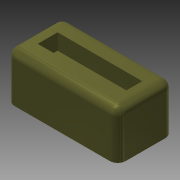
# Autodesk Inventor part: cover
Saved by Autodesk Inventor 2014 SP1 (Build 180222100, 222)
## iProperties
Created: 2016-10-06
Part Number: cover
Material: Titanium
Document SubType Name: Modeling
Designer: tguillod
Density: 4.51 g/cm^3
Appearance: Titanium
Author: tguillod
Autodesk Inventor part; units mm, degrees
ref_plane "YZ Plane" through (0, 0, 0) normal (1, 0, 0) x (0, 1, 0)
ref_plane "XZ Plane" through (0, 0, 0) normal (0, 1, 0) x (-1, 0, 0)
ref_plane "XY Plane" through (0, 0, 0) normal (0, 0, 1) x (1, 0, 0)
sketch "Sketch1" plane through (0, 0, 0) normal (0, 0, 1) x (1, 0, 0)
  line L0 (0, 0) -> (14, 0)
  line L1 (14, 0) -> (14, 7)
  line L2 (14, 7) -> (0, 7)
  line L3 (0, 7) -> (0, 0)
  dimension "d2" = 14
  dimension "d3" = 7
  constraints: 8 end point, 2 parallel, 1 horizontal, 1 perpendicular
  measures "d2" distance of L1.end L2.end
  measures "d3" distance of L0.end L1.end
extrude "Extrusion1" add sketch "Sketch1" along normal blind 6
sketch "Sketch2" plane through (0, 0, 6) normal (0, 0, 1) x (1, 0, 0)
  line L0 (0, 7) -> (14, 0) construction
  line L1 (0, 0) -> (14, 7) construction
  line L2 (1.67, 4.75) -> (12.33, 4.75)
  line L3 (12.33, 4.75) -> (12.33, 2.25)
  line L4 (12.33, 2.25) -> (1.67, 2.25)
  line L5 (1.67, 2.25) -> (1.67, 4.75)
  line L6 (1.67, 4.75) -> (12.33, 2.25) construction
  line L7 (12.33, 4.75) -> (1.67, 2.25) construction
  point P0 (7, 3.5)
  dimension "d4" = 2.5
  dimension "d5" = 10.66
  constraints: 16 end point, 3 midpoint, 2 parallel, 1 horizontal, 1 perpendicular
  measures "d4" distance of L2.end L3.end
  measures "d5" distance of L2.start L2.end
extrude "Extrusion3" cut sketch "Sketch2" against normal blind 2
sketch "Sketch3" plane through (0, 0, 4) normal (0, 0, 1) x (1, 0, 0)
  line L0 (1.67, 4.75) -> (12.33, 4.75) projected
  line L1 (1.67, 2.25) -> (1.67, 4.75) projected
  line L2 (12.33, 2.25) -> (1.67, 2.25) projected
  line L3 (12.33, 4.75) -> (12.33, 2.25) projected
  line L4 (2.67, 3.75) -> (11.33, 3.75)
  line L5 (11.33, 3.75) -> (11.33, 3.25)
  line L6 (11.33, 3.25) -> (2.67, 3.25)
  line L7 (2.67, 3.25) -> (2.67, 3.75)
  point P0 (0, 0)
  dimension "d10" = 1
  dimension "d11" = 1
  dimension "d12" = 1
  dimension "d13" = 1
  constraints: 8 end point, 2 parallel, 1 horizontal, 1 perpendicular
  measures "d10" distance between parallel lines of L1 L7
  measures "d11" distance between parallel lines of L3 L5
  measures "d12" distance between parallel lines of L0 L4
  measures "d13" distance between parallel lines of L6 L2
extrude "Extrusion4" cut sketch "Sketch3" against normal blind 4 contours L4 L5 L6 L7
sketch "Sketch4" plane through (0, 0, 0) normal (0, 0, -1) x (-1, 0, 0)
  line L0 (-2.67, 3.75) -> (-2.67, 3.25) projected
  line L1 (-2.67, 3.25) -> (-11.33, 3.25) projected
  line L2 (-11.33, 3.25) -> (-11.33, 3.75) projected
  line L3 (-11.33, 3.75) -> (-2.67, 3.75) projected
  line L4 (0, 0) -> (-14, 0) projected
  line L5 (0, 7) -> (0, 0) projected
  line L6 (-14, 7) -> (0, 7) projected
  line L7 (-14, 0) -> (-14, 7) projected
  line L8 (-13, 6) -> (-1, 6)
  line L9 (-1, 6) -> (-1, 1)
  line L10 (-1, 1) -> (-13, 1)
  line L11 (-13, 1) -> (-13, 6)
  dimension "d16" = 1
  dimension "d17" = 1
  dimension "d18" = 1
  dimension "d19" = 1
  constraints: 8 end point, 2 parallel, 1 horizontal, 1 perpendicular
  measures "d16" distance between parallel lines of L6 L8
  measures "d17" distance between parallel lines of L10 L4
  measures "d18" distance between parallel lines of L11 L7
  measures "d19" distance between parallel lines of L5 L9
extrude "Extrusion5" cut sketch "Sketch4" against normal blind 3 contours L8 L9 L10 L11
sketch "Sketch5" plane through (0, 7, 0) normal (0, 1, 0) x (1, 0, 0)
  line L0 (14, 0) -> (0, 0) projected
  line L1 (0, 0) -> (0, -6) projected
  line L2 (14, 0) -> (14, -6) projected
  line L3 (5.5, 0) -> (8.5, 0)
  line L4 (8.5, 0) -> (8.5, -1)
  line L5 (8.5, -1) -> (5.5, -1)
  line L6 (5.5, -1) -> (5.5, 0)
  dimension "d22" = 1
  dimension "d23" = 5.5
  dimension "d24" = 5.5
  dimension "d25" = 3
  constraints: 8 end point, 2 parallel, 1 horizontal, 1 perpendicular, 1 point on line
  measures "d22" distance of L3.end L4.end
  measures "d23" distance between parallel lines of L2 L4
  measures "d24" distance between parallel lines of L1 L6
  measures "d25" distance of L4.end L5.end
extrude "Extrusion6" cut sketch "Sketch5" against normal blind 1
fillet "Fillet1" radius 1 8 edges at (7, 0, 6) (14, 3.5, 6) (14, 0, 3) (7, 7, 6) (14, 7, 3) (0, 0, 3) (0, 3.5, 6) (0, 7, 3)
body "Solid1"
